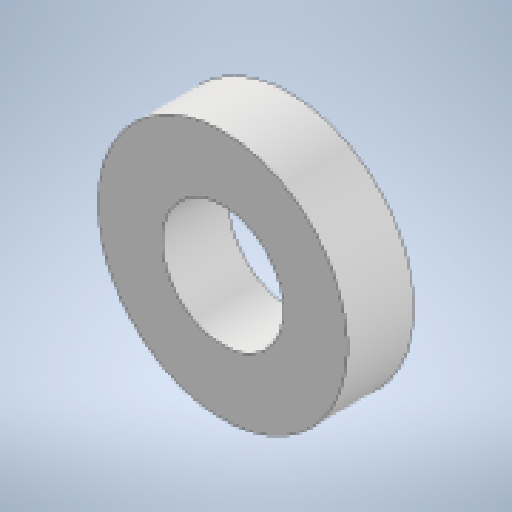
# Autodesk Inventor part: 100spacer
Saved by Autodesk Inventor 2023 (Build 270158000, 158)
## iProperties
Created: 2022-11-11
Part Number: 100spacer
Material: Generic
Document SubType Name: Modeling
Designer: Zac Hah
Density: 1 g/cm^3
Appearance: Default
Author: Zac Hah
Autodesk Inventor part; units mm, degrees
ref_plane "YZ Plane" through (0, 0, 0) normal (1, 0, 0) x (0, 1, 0)
ref_plane "XZ Plane" through (0, 0, 0) normal (0, 1, 0) x (-1, 0, 0)
ref_plane "XY Plane" through (0, 0, 0) normal (0, 0, 1) x (1, 0, 0)
sketch "Sketch1" plane through (0, 0, 0) normal (0, 0, 1) x (1, 0, 0)
  line L0 (-1.6002, 1.6002) -> (1.6002, 1.6002)
  line L1 (1.6002, 1.6002) -> (1.6002, -1.6002)
  line L2 (1.6002, -1.6002) -> (-1.6002, -1.6002)
  line L3 (-1.6002, -1.6002) -> (-1.6002, 1.6002)
  line L4 (-1.6002, 1.6002) -> (1.6002, -1.6002) construction
  line L5 (1.6002, 1.6002) -> (-1.6002, -1.6002) construction
  circle A0 centre (0, 0) radius 2.3114
  circle A1 centre (0, 0) radius 4.7625
  dimension "d0" = 3.2004
  dimension "d1" = 3.2004
  dimension "d2" = 4.6228
  dimension "d3" = 9.525
  constraints: 12 end point, 2 centre point, 2 coincident, 2 midpoint, 2 parallel, 1 horizontal, 1 perpendicular
  measures "d0" distance of L1.end L2.end
  measures "d1" distance of L0.end L1.end
  measures "d2" diameter of A0
  measures "d3" diameter of A1
extrude "Extrusion1" add sketch "Sketch1" along normal blind 2.54 contours A1
body "Solid1"
